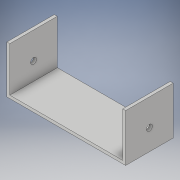
# Autodesk Inventor part: ScissorLIftBracketOutside
Saved by Autodesk Inventor 2018 (Build 220112000, 112)
## iProperties
Created: 2020-01-25
Part Number: ScissorLIftBracketOutside
Material: Generic
Document SubType Name: Modeling
Designer: Cooper
Density: 1 g/cm^3
Appearance: Default
Author: Cooper
Autodesk Inventor part; units mm, degrees
ref_plane "YZ Plane" through (0, 0, 0) normal (1, 0, 0) x (0, 1, 0)
ref_plane "XZ Plane" through (0, 0, 0) normal (0, 1, 0) x (-1, 0, 0)
ref_plane "XY Plane" through (0, 0, 0) normal (0, 0, 1) x (1, 0, 0)
sketch "Sketch1" plane through (0, 0, 0) normal (0, 0, 1) x (1, 0, 0)
  line L0 (0, 0) -> (0, 50.8)
  line L1 (0, 50.8) -> (3.175, 50.8)
  line L2 (3.175, 50.8) -> (3.175, 3.175)
  line L3 (3.175, 3.175) -> (123.825, 3.175)
  line L4 (123.825, 3.175) -> (123.825, 50.8)
  line L5 (123.825, 50.8) -> (127, 50.8)
  line L6 (127, 50.8) -> (127, 0)
  line L7 (127, 0) -> (0, 0)
  dimension "d0" = 3.175
  dimension "d2" = 3.175
  dimension "d3" = 3.175
  dimension "d4" = 127
  dimension "d5" = 50.8
  constraints: 16 end point, 3 vertical, 2 horizontal, 2 perpendicular, 1 parallel, 1 point on line
  measures "d0" distance between parallel lines of L2 L0
  measures "d2" distance between parallel lines of L6 L4
  measures "d3" distance between parallel lines of L7 L3
  measures "d4" distance of L6.end L0.start
  measures "d5" distance of L0.start L0.end
extrude "Extrusion1" add sketch "Sketch1" along normal blind 50.8
sketch "Sketch2" plane through (127, 0, 0) normal (1, 0, 0) x (0, 0, -1)
  line L0 (0, 50.8) -> (0, 0) projected
  line L1 (0, 50.8) -> (-50.8, 50.8) projected
  line L2 (-50.8, 0) -> (-50.8, 50.8) projected
  line L3 (0, 0) -> (-50.8, 0) projected
  point P0 (0, 0)
  point P1 (-25.4, 22.225)
  dimension "d8" = 25.4
  dimension "d9" = 25.4
  dimension "d10" = 22.225
  measures "d8" distance from line of point (-25.4, 22.225) L2
  measures "d9" distance from line of L0 point (-25.4, 22.225)
  measures "d10" distance from line of L3 point (-25.4, 22.225)
hole "Hole1" at (127, 22.225, 25.4) direction (-1, 0, 0) diameter 6.35 end through all
equation "\"d2\" = d0"
equation "\"d3\" = d0"
equation "\"d8\" = d9"
body "Solid1"
